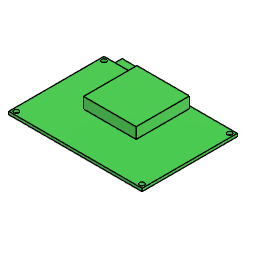
Fusion_360_projekt_ohišje (Autodesk Fusion 360 archive; units mm, degrees)
design "pcb1"
Autodesk Fusion 360 part; units mm, degrees
sketch "Sketch2" plane through (0, 0, 0) normal (0, 0, 1) x (1, 0, 0)
  line L0 (0, 0) -> (70, 0)
  line L1 (70, 0) -> (70, 50)
  line L2 (70, 50) -> (0, 50)
  line L3 (0, 50) -> (0, 0)
  dimension "d1" = 70
  dimension "d2" = 50
  constraint horizontal L0
  constraint vertical L1
  constraint horizontal L2
  constraint vertical L3
  constraint coincident L0.start L3.end
  measures "d1" distance of L0.start L0.end
  measures "d2" distance of L0.start L2.end
extrude "Extrude1" add sketch "Sketch2" along normal blind 1.5
sketch "Sketch3" plane through (0, 0, 1.5) normal (0, 0, 1) x (-1, 0, 0)
  line L0 (0, -50) -> (0, 0)
  line L1 (0, 0) -> (-70, 0)
  line L2 (-70, 0) -> (-70, -50)
  line L3 (-70, -50) -> (0, -50)
  line L4 (-18.6, -48.7) -> (-46.2, -48.7)
  line L5 (-46.2, -48.7) -> (-46.2, -20.7)
  line L6 (-46.2, -20.7) -> (-18.6, -20.7)
  line L7 (-18.6, -20.7) -> (-18.6, -48.7)
  line L8 (-28, -48.7) -> (-28, -50) construction
  line L9 (-18.6, -42) -> (0, -42) construction
  dimension "d5" = 27.6
  dimension "d6" = 28
  dimension "d7" = 1.3
  dimension "d8" = 18.6
  constraint horizontal L4
  constraint vertical L5
  constraint horizontal L6
  constraint vertical L7
  constraint coincident L4 L8.start
  constraint coincident L3 L8.end
  constraint perpendicular L3 L8
  constraint coincident L7 L9.start
  constraint coincident L0 L9.end
  constraint perpendicular L0 L9
  measures "d5" distance of L4.start L4.end
  measures "d6" distance of L4.start L6.end
  measures "d7" distance of L8.start L8.end
  measures "d8" distance of L9.start L9.end
extrude "Extrude2" add sketch "Sketch3" along normal blind 5.75 contours L4 L5 L6 L7
sketch "Sketch4" plane through (0, 0, 0) normal (0, 0, -1) x (1, 0, 0)
  line L0 (0, 0) -> (0, -50)
  line L1 (0, -50) -> (70, -50)
  line L2 (70, -50) -> (70, 0)
  line L3 (70, 0) -> (0, 0)
  line L4 (4.3, -21) -> (27.8, -21)
  line L5 (27.8, -21) -> (27.8, -55.25)
  line L6 (27.8, -55.25) -> (4.3, -55.25)
  line L7 (4.3, -55.25) -> (4.3, -21)
  dimension "d11" = 23.5
  dimension "d12" = 34.25
  dimension "d17" = 5.25
  dimension "d18" = 4.3
  constraint horizontal L4
  constraint vertical L5
  constraint horizontal L6
  constraint vertical L7
  measures "d11" distance of L4.start L4.end
  measures "d12" distance of L4.start L6.end
  measures "d17" distance of L1 L6
  measures "d18" distance of L0 L7
extrude "Extrude3" add sketch "Sketch4" along normal blind 12 contours L1 L4 L5 L7 | L1 L5 L6 L7
sketch "Sketch5" plane through (0, 0, 1.5) normal (0, 0, 1) x (-1, 0, 0)
  line L0 (-18.6, -20.7) -> (-18.6, -48.7)
  line L1 (-18.6, -48.7) -> (-46.2, -48.7)
  line L2 (-46.2, -48.7) -> (-46.2, -20.7)
  line L3 (-46.2, -20.7) -> (-18.6, -20.7)
  line L4 (0, -50) -> (0, 0)
  line L5 (0, 0) -> (-70, 0)
  line L6 (-70, 0) -> (-70, -50)
  line L7 (-70, -50) -> (0, -50)
  line L8 (-2, -50) -> (-2, -48) construction
  line L9 (0, -48) -> (-2, -48) construction
  circle A0 centre (-2, -48) radius 1.25
  line L10 (-2, 0) -> (-2, -2) construction
  line L11 (0, -2) -> (-2, -2) construction
  circle A1 centre (-2, -2) radius 1.25
  line L12 (-70, -2) -> (-68, -2) construction
  line L13 (-68, -2) -> (-68, 0) construction
  circle A2 centre (-68, -2) radius 1.25
  line L14 (-68, -50) -> (-68, -48) construction
  line L15 (-68, -48) -> (-70, -48) construction
  circle A3 centre (-68, -48) radius 1.25
  dimension "d21" = 2
  dimension "d22" = 2
  dimension "d23" = 2.5
  dimension "d24" = 2
  dimension "d25" = 2
  dimension "d26" = 2.5
  dimension "d27" = 2
  dimension "d28" = 2
  dimension "d29" = 2.5
  dimension "d30" = 2
  dimension "d31" = 2
  dimension "d32" = 2.5
  constraint coincident L7 L8.start
  constraint perpendicular L7 L8
  constraint coincident L4 L9.start
  constraint coincident L8.end L9.end
  constraint coincident L5 L10.start
  constraint perpendicular L5 L10
  constraint coincident L4 L11.start
  constraint coincident L10.end L11.end
  constraint coincident L6 L12.start
  constraint perpendicular L6 L12
  constraint coincident L5 L13.end
  constraint perpendicular L5 L13
  constraint coincident L12.end L13.start
  constraint coincident L7 L14.start
  constraint perpendicular L7 L14
  constraint coincident L6 L15.end
  constraint perpendicular L6 L15
  constraint coincident L14.end L15.start
  measures "d21" distance of L8.start L8.end
  measures "d22" distance of L8.end L9.start
  measures "d23" diameter of A0
  measures "d24" distance of L10.start L10.end
  measures "d25" distance of L10.end L11.start
  measures "d26" diameter of A1
  measures "d27" distance of L12.start L12.end
  measures "d28" distance of L12.end L13.end
  measures "d29" diameter of A2
  measures "d30" distance of L14.start L14.end
  measures "d31" distance of L14.end L15.end
  measures "d32" diameter of A3
extrude "Extrude4" cut sketch "Sketch5" against normal up to surface (1.5 mm away) contours A0 | A1 | A2 | A3

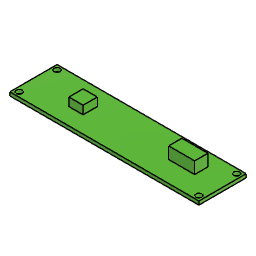
design "pcb2"
Autodesk Fusion 360 part; units mm, degrees
sketch "Sketch1" plane through (0, 0, 0) normal (0, 0, 1) x (1, 0, 0)
  line L0 (0, 0) -> (80, 0)
  line L1 (80, 0) -> (80, 20)
  line L2 (80, 20) -> (0, 20)
  line L3 (0, 20) -> (0, 0)
  line L4 (2, 20) -> (2, 18) construction
  line L5 (0, 18) -> (2, 18) construction
  circle A0 centre (2, 18) radius 1.25
  line L6 (78, 20) -> (78, 18) construction
  line L7 (80, 17.9933) -> (78, 18) construction
  circle A1 centre (78, 18) radius 1.25
  line L8 (80, 2) -> (78, 2) construction
  line L9 (78, 0) -> (78, 2) construction
  circle A2 centre (78, 2) radius 1.25
  line L10 (0, 2) -> (2, 2) construction
  line L11 (2, 0) -> (2, 2) construction
  circle A3 centre (2, 2) radius 1.25
  dimension "d1" = 80
  dimension "d2" = 20
  dimension "d5" = 2
  dimension "d6" = 2
  dimension "d7" = 2.5
  dimension "d8" = 2
  dimension "d9" = 2
  dimension "d10" = 2.5
  dimension "d13" = 2
  dimension "d14" = 2
  dimension "d15" = 2.5
  dimension "d16" = 2
  dimension "d17" = 2
  dimension "d18" = 2.5
  constraint horizontal L0
  constraint vertical L1
  constraint horizontal L2
  constraint vertical L3
  constraint coincident L0.start L3.end
  constraint coincident L2 L4.start
  constraint perpendicular L2 L4
  constraint coincident L3 L5.start
  constraint coincident L4.end L5.end
  constraint coincident L2 L6.start
  constraint perpendicular L2 L6
  constraint coincident L1 L7.start
  constraint coincident L6.end L7.end
  constraint coincident L1 L8.start
  constraint perpendicular L1 L8
  constraint coincident L0 L9.start
  constraint coincident L8.end L9.end
  constraint coincident L3 L10.start
  constraint perpendicular L3 L10
  constraint coincident L0 L11.start
  constraint coincident L10.end L11.end
  measures "d1" distance of L0.start L0.end
  measures "d2" distance of L0.start L2.end
  measures "d5" distance of L4.start L4.end
  measures "d6" distance of L4.end L5.start
  measures "d7" diameter of A0
  measures "d8" distance of L6.start L6.end
  measures "d9" horizontal distance of L6.end L7.start
  measures "d10" diameter of A1
  measures "d13" distance of L8.start L8.end
  measures "d14" distance of L8.end L9.start
  measures "d15" diameter of A2
  measures "d16" distance of L10.start L10.end
  measures "d17" distance of L10.end L11.start
  measures "d18" diameter of A3
extrude "Extrude2" add sketch "Sketch1" along normal blind 1.5
sketch "Sketch2" plane through (0, 0, 1.5) normal (0, 0, 1) x (-1, 0, 0)
  circle A0 centre (-2, -18) radius 1.25
  circle A1 centre (-78, -2) radius 1.25
  circle A2 centre (-78, -18) radius 1.25
  circle A3 centre (-2, -2) radius 1.25
  line L0 (0, -20) -> (0, 0)
  line L1 (0, 0) -> (-80, 0)
  line L2 (-80, 0) -> (-80, -20)
  line L3 (-80, -20) -> (0, -20)
  line L4 (-17.9, -13.1) -> (-23.9, -13.1)
  line L5 (-23.9, -13.1) -> (-23.9, -7.1)
  line L6 (-23.9, -7.1) -> (-17.9, -7.1)
  line L7 (-17.9, -7.1) -> (-17.9, -13.1)
  line L8 (-20.9, -20) -> (-20.9, -13.1) construction
  line L9 (0, -11) -> (-17.9, -11) construction
  line L10 (-58.4, -14.4) -> (-69.4, -14.4)
  line L11 (-69.4, -14.4) -> (-69.4, -8.8)
  line L12 (-69.4, -8.8) -> (-58.4, -8.8)
  line L13 (-58.4, -8.8) -> (-58.4, -14.4)
  line L14 (-64.8436, -20) -> (-64.8436, -14.4) construction
  line L15 (-69.4, -11.6) -> (-80, -11.6) construction
  dimension "d21" = 6
  dimension "d22" = 6
  dimension "d23" = 6.9
  dimension "d26" = 17.9
  dimension "d27" = 11
  dimension "d28" = 5.6
  dimension "d29" = 5.6
  dimension "d30" = 10.6
  constraint horizontal L4
  constraint vertical L5
  constraint horizontal L6
  constraint vertical L7
  constraint coincident L3 L8.start
  constraint midpoint L4 L8.end
  constraint coincident L0 L9.start
  constraint coincident L7 L9.end
  constraint perpendicular L7 L9
  constraint horizontal L10
  constraint vertical L11
  constraint horizontal L12
  constraint vertical L13
  constraint coincident L3 L14.start
  constraint coincident L10 L14.end
  constraint perpendicular L10 L14
  constraint midpoint L11 L15.start
  constraint coincident L2 L15.end
  constraint perpendicular L2 L15
  measures "d21" distance of L4.start L4.end
  measures "d22" distance of L4.start L6.end
  measures "d23" vertical distance of L8.start L8.end
  measures "d26" distance of L9.start L9.end
  measures "d27" distance of L10.start L10.end
  measures "d28" distance of L10.start L12.end
  measures "d29" distance of L14.start L14.end
  measures "d30" distance of L15.start L15.end
extrude "Extrude3" add sketch "Sketch2" along normal blind 5 contours L10 L11 L12 L13
extrude "Extrude4" add sketch "Sketch2" along normal blind 3.5 contours L4 L5 L6 L7
